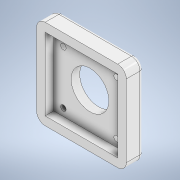
# Autodesk Inventor part: motor mount
Saved by Autodesk Inventor 2020 (Build 240168000, 168)
## iProperties
Created: 2021-03-03
Part Number: motor mount
Material: ABS Plastic
Document SubType Name: Modeling
Designer: AOB
Mass: 16.9182 g
Surface Area: 78.2786 cm^2
Volume: 15.9605 cm^3
Density: 1.06 g/cm^3
Appearance: White
Author: AOB
Autodesk Inventor part; units mm, degrees
ref_plane "YZ Plane" through (0, 0, 0) normal (1, 0, 0) x (0, 1, 0)
ref_plane "XZ Plane" through (0, 0, 0) normal (0, 1, 0) x (-1, 0, 0)
ref_plane "XY Plane" through (0, 0, 0) normal (0, 0, 1) x (1, 0, 0)
sketch "Sketch1" plane through (0, 0, 0) normal (0, 0, 1) x (1, 0, 0)
  line L0 (0, 0) -> (42.3, 0)
  line L1 (42.3, 0) -> (42.3, -42.3)
  line L2 (42.3, -42.3) -> (0, -42.3)
  line L3 (0, -42.3) -> (0, 0)
  line L4 (0, 5) -> (-5, 5)
  line L5 (-5, 5) -> (47.3, 5)
  line L6 (47.3, 5) -> (47.3, -47.3)
  line L7 (47.3, -47.3) -> (-5, -47.3)
  line L8 (-5, -47.3) -> (-5, 5)
  line L9 (21.15, -15.5) -> (5.65, -15.5) construction
  line L10 (5.65, -22.5) -> (5.65, -7) construction
  line L11 (5.65, -7) -> (36.65, -7) construction
  line L12 (36.65, -7) -> (36.65, -38) construction
  line L13 (36.65, -38) -> (5.65, -38) construction
  line L14 (42.3, 0) -> (0, -42.3) construction
  line L15 (0, 0) -> (21.15, -21.15) construction
  dimension "d1" = 42.3
  dimension "d3" = 5
  dimension "d4" = 52.3
  dimension "d5" = 52.3
  dimension "d7" = 15.5
  dimension "d8" = 15.5
  dimension "d9" = 31
  dimension "d10" = 31
  constraints: 32 end point, 5 perpendicular, 4 parallel, 2 horizontal, 1 midpoint, 1 point on line, 1 vertical
  measures "d1" distance of L0.end L1.end
  measures "d3" distance of L0.start L4.start
  measures "d4" distance of L6.end L7.end
  measures "d5" distance of L7.end L4.end
  measures "d7" distance of L9.start L9.end
  measures "d8" distance of L10.start L10.end
  measures "d9" distance of L10.end L11.end
  measures "d10" distance of L11.end L12.end
extrude "Extrusion1" add sketch "Sketch1" along normal blind 5
extrude "Extrusion2" add sketch "Sketch1" against normal blind 5 contours L0 L1 L2 L3 | L5 L6 L7 L8 L4
hole "Hole1" at (5.65, -7, 0) at (36.65, -7, 0) at (36.65, -38, 0) at (5.65, -38, 0) direction (0, 0, -1) diameter 3.2 end through all
fillet "Fillet4" radius 5 4 edges at (47.3, 5, 0) (47.3, -47.3, 0) (-5, 5, 0) (-5, -47.3, 0)
fillet "Fillet5" radius 2 8 edges at (45.8355, 3.5355, -5) (47.3, -21.15, -5) (45.8355, -45.8355, -5) (21.15, -47.3, -5) (-3.5355, -45.8355, -5) (-5, -21.15, -5) (-3.5355, 3.5355, -5) (21.15, 5, -5)
hole "Hole2" at (21.15, -21.15, 0) direction (0, 0, -1) diameter 22 end through all
body "Solid1"
